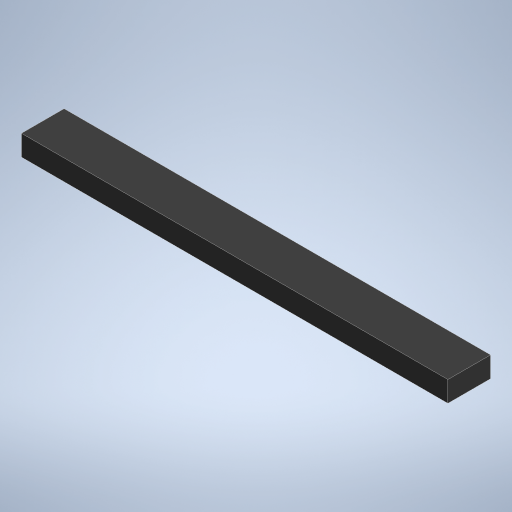
# Autodesk Inventor part: Board connector
Saved by Autodesk Inventor 2023 (Build 270158000, 158)
## iProperties
Created: 2022-12-30
Part Number: Board connector
Material: Generico
Document SubType Name: Modeling
Designer: Gabriele
Density: 1 g/cm^3
Appearance: Gomma - Nero
Author: Gabriele
Autodesk Inventor part; units mm, degrees
ref_plane "YZ Plane" through (0, 0, 0) normal (1, 0, 0) x (0, 1, 0)
ref_plane "XZ Plane" through (0, 0, 0) normal (0, 1, 0) x (-1, 0, 0)
ref_plane "XY Plane" through (0, 0, 0) normal (0, 0, 1) x (1, 0, 0)
sketch "Schizzo1" plane through (0, 0, 0) normal (0, 0, 1) x (1, 0, 0)
  line L0 (-30, -1.45) -> (30, -1.45)
  line L1 (30, -1.45) -> (30, 1.45)
  line L2 (30, 1.45) -> (-30, 1.45)
  line L3 (-30, 1.45) -> (-30, -1.45)
  line L4 (-30, -1.45) -> (30, 1.45) construction
  line L5 (30, -1.45) -> (-30, 1.45) construction
  point P0 (0, 0)
  dimension "d0" = 60
  dimension "d1" = 2.9
  constraints: 12 end point, 2 midpoint, 2 parallel, 1 horizontal, 1 perpendicular
  measures "d0" distance of L1.end L2.end
  measures "d1" distance of L0.end L1.end
extrude "Estrusione1" add sketch "Schizzo1" along normal blind 6
